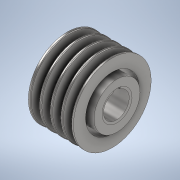
# Autodesk Inventor part: Polia Motora 3D
Saved by Autodesk Inventor 2021 (Build 250183000, 183)
## iProperties
Created: 2021-03-22
Part Number: Polia Motora 3D
Material: Steel, Carbon
Document SubType Name: Modeling
Designer: mathe
Mass: 3334.35 g
Surface Area: 1037.05 cm^2
Volume: 424.758 cm^3
Density: 7.85 g/cm^3
Appearance: Semi-Polished
Author: mathe
Autodesk Inventor part; units mm, degrees
ref_plane "YZ Plane" through (0, 0, 0) normal (1, 0, 0) x (0, 1, 0)
ref_plane "XZ Plane" through (0, 0, 0) normal (0, 1, 0) x (-1, 0, 0)
ref_plane "XY Plane" through (0, 0, 0) normal (0, 0, 1) x (1, 0, 0)
sketch "Sketch1" plane through (0, 0, 0) normal (0, 0, 1) x (1, 0, 0)
  arc A0 (466.2251, 430.0149) -> (467.1814, 430.7225) centre (466.2251, 431.0149) ccw
  arc A1 (466.2251, 430.0149) -> (467.1814, 430.7225) centre (466.2251, 431.0149) ccw
  arc A2 (478.0277, 430.7225) -> (478.984, 430.0149) centre (478.984, 431.0149) ccw
  arc A3 (478.0277, 430.7225) -> (478.984, 430.0149) centre (478.984, 431.0149) ccw
  line L0 (478.984, 430.0149) -> (482.1051, 430.0149)
  line L1 (478.984, 430.0149) -> (482.1051, 430.0149)
  line L2 (463.104, 430.0149) -> (466.2251, 430.0149)
  line L3 (463.104, 430.0149) -> (466.2251, 430.0149)
  arc A4 (482.1051, 430.0149) -> (483.0614, 430.7225) centre (482.1051, 431.0149) ccw
  arc A5 (482.1051, 430.0149) -> (483.0614, 430.7225) centre (482.1051, 431.0149) ccw
  arc A6 (462.1477, 430.7225) -> (463.104, 430.0149) centre (463.104, 431.0149) ccw
  arc A7 (462.1477, 430.7225) -> (463.104, 430.0149) centre (463.104, 431.0149) ccw
  line L4 (490.0745, 430.0149) -> (490.0745, 425.0149)
  line L5 (490.0745, 425.0149) -> (461.1309, 425.0149)
  line L6 (490.0745, 443.0149) -> (490.0745, 430.0149)
  line L7 (487.5595, 443.0149) -> (490.0745, 443.0149)
  line L8 (487.5595, 443.0149) -> (490.0745, 443.0149)
  line L9 (486.6032, 442.3073) -> (483.0614, 430.7225)
  line L10 (486.6032, 442.3073) -> (483.0614, 430.7225)
  line L11 (474.4859, 442.3073) -> (478.0277, 430.7225)
  line L12 (474.4859, 442.3073) -> (478.0277, 430.7225)
  line L13 (470.7232, 442.3073) -> (467.1814, 430.7225)
  line L14 (470.7232, 442.3073) -> (467.1814, 430.7225)
  arc A8 (471.6795, 443.0149) -> (470.7232, 442.3073) centre (471.6795, 442.0149) ccw
  arc A9 (471.6795, 443.0149) -> (470.7232, 442.3073) centre (471.6795, 442.0149) ccw
  line L15 (471.6795, 443.0149) -> (473.5296, 443.0149)
  line L16 (471.6795, 443.0149) -> (473.5296, 443.0149)
  arc A10 (474.4859, 442.3073) -> (473.5296, 443.0149) centre (473.5296, 442.0149) ccw
  arc A11 (474.4859, 442.3073) -> (473.5296, 443.0149) centre (473.5296, 442.0149) ccw
  arc A12 (453.1309, 419.5149) -> (454.1309, 420.5149) centre (453.1309, 420.5149) ccw
  arc A13 (460.1309, 420.5149) -> (461.1309, 419.5149) centre (461.1309, 420.5149) ccw
  line L17 (454.1309, 424.0149) -> (454.1309, 420.5149)
  arc A14 (461.1309, 425.0149) -> (460.1309, 424.0149) centre (461.1309, 424.0149) ccw
  arc A15 (454.1309, 424.0149) -> (453.1309, 425.0149) centre (453.1309, 424.0149) ccw
  line L18 (418.1309, 404.5149) -> (417.1309, 407.7149)
  line L19 (417.1309, 419.5149) -> (453.1309, 419.5149)
  line L20 (453.1309, 425.0149) -> (423.3745, 425.0149)
  arc A16 (434.4651, 430.0149) -> (435.4214, 430.7225) centre (434.4651, 431.0149) ccw
  arc A17 (434.4651, 430.0149) -> (435.4214, 430.7225) centre (434.4651, 431.0149) ccw
  arc A18 (430.3877, 430.7225) -> (431.344, 430.0149) centre (431.344, 431.0149) ccw
  arc A19 (430.3877, 430.7225) -> (431.344, 430.0149) centre (431.344, 431.0149) ccw
  line L21 (460.1309, 420.5149) -> (460.1309, 424.0149)
  line L22 (490.0745, 341.0149) -> (490.0745, 346.0149)
  line L23 (490.0745, 328.0149) -> (490.0745, 341.0149)
  arc A20 (483.0614, 340.3073) -> (482.1051, 341.0149) centre (482.1051, 340.0149) ccw
  arc A21 (483.0614, 340.3073) -> (482.1051, 341.0149) centre (482.1051, 340.0149) ccw
  line L24 (487.5595, 328.0149) -> (490.0745, 328.0149)
  line L25 (487.5595, 328.0149) -> (490.0745, 328.0149)
  arc A22 (486.6032, 328.7225) -> (487.5595, 328.0149) centre (487.5595, 329.0149) ccw
  arc A23 (486.6032, 328.7225) -> (487.5595, 328.0149) centre (487.5595, 329.0149) ccw
  line L26 (478.984, 341.0149) -> (482.1051, 341.0149)
  line L27 (478.984, 341.0149) -> (482.1051, 341.0149)
  arc A24 (478.984, 341.0149) -> (478.0277, 340.3073) centre (478.984, 340.0149) ccw
  arc A25 (478.984, 341.0149) -> (478.0277, 340.3073) centre (478.984, 340.0149) ccw
  line L28 (486.6032, 328.7225) -> (483.0614, 340.3073)
  line L29 (486.6032, 328.7225) -> (483.0614, 340.3073)
  line L30 (474.4859, 328.7225) -> (478.0277, 340.3073)
  line L31 (474.4859, 328.7225) -> (478.0277, 340.3073)
  arc A26 (473.5296, 328.0149) -> (474.4859, 328.7225) centre (473.5296, 329.0149) ccw
  arc A27 (473.5296, 328.0149) -> (474.4859, 328.7225) centre (473.5296, 329.0149) ccw
  line L32 (471.6795, 328.0149) -> (473.5296, 328.0149)
  line L33 (471.6795, 328.0149) -> (473.5296, 328.0149)
  arc A28 (470.7232, 328.7225) -> (471.6795, 328.0149) centre (471.6795, 329.0149) ccw
  arc A29 (470.7232, 328.7225) -> (471.6795, 328.0149) centre (471.6795, 329.0149) ccw
  line L34 (490.0745, 346.0149) -> (461.1309, 346.0149)
  line L35 (460.1309, 350.5149) -> (460.1309, 347.0149)
  arc A30 (460.1309, 347.0149) -> (461.1309, 346.0149) centre (461.1309, 347.0149) ccw
  line L36 (461.1309, 351.5149) -> (497.1309, 351.5149)
  arc A31 (453.1309, 346.0149) -> (454.1309, 347.0149) centre (453.1309, 347.0149) ccw
  arc A32 (438.9632, 328.7225) -> (439.9195, 328.0149) centre (439.9195, 329.0149) ccw
  arc A33 (438.9632, 328.7225) -> (439.9195, 328.0149) centre (439.9195, 329.0149) ccw
  line L37 (439.9195, 328.0149) -> (441.7696, 328.0149)
  line L38 (439.9195, 328.0149) -> (441.7696, 328.0149)
  arc A34 (441.7696, 328.0149) -> (442.7259, 328.7225) centre (441.7696, 329.0149) ccw
  arc A35 (441.7696, 328.0149) -> (442.7259, 328.7225) centre (441.7696, 329.0149) ccw
  line L39 (442.7259, 328.7225) -> (446.2677, 340.3073)
  arc A36 (447.224, 341.0149) -> (446.2677, 340.3073) centre (447.224, 340.0149) ccw
  arc A37 (447.224, 341.0149) -> (446.2677, 340.3073) centre (447.224, 340.0149) ccw
  line L40 (447.224, 341.0149) -> (450.3451, 341.0149)
  line L41 (447.224, 341.0149) -> (450.3451, 341.0149)
  arc A38 (451.3014, 340.3073) -> (450.3451, 341.0149) centre (450.3451, 340.0149) ccw
  arc A39 (451.3014, 340.3073) -> (450.3451, 341.0149) centre (450.3451, 340.0149) ccw
  line L42 (454.1309, 347.0149) -> (454.1309, 350.5149)
  line L43 (454.8432, 328.7225) -> (451.3014, 340.3073)
  line L44 (454.8432, 328.7225) -> (451.3014, 340.3073)
  line L45 (442.7259, 328.7225) -> (446.2677, 340.3073)
  line L46 (453.1309, 346.0149) -> (423.3745, 346.0149)
  line L47 (438.9632, 328.7225) -> (435.4214, 340.3073)
  line L48 (438.9632, 328.7225) -> (435.4214, 340.3073)
  arc A40 (435.4214, 340.3073) -> (434.4651, 341.0149) centre (434.4651, 340.0149) ccw
  line L49 (431.344, 341.0149) -> (434.4651, 341.0149)
  line L50 (431.344, 341.0149) -> (434.4651, 341.0149)
  arc A41 (431.344, 341.0149) -> (430.3877, 340.3073) centre (431.344, 340.0149) ccw
  arc A42 (431.344, 341.0149) -> (430.3877, 340.3073) centre (431.344, 340.0149) ccw
  line L51 (426.8459, 328.7225) -> (430.3877, 340.3073)
  line L52 (426.8459, 328.7225) -> (430.3877, 340.3073)
  arc A43 (425.8896, 328.0149) -> (426.8459, 328.7225) centre (425.8896, 329.0149) ccw
  arc A44 (425.8896, 328.0149) -> (426.8459, 328.7225) centre (425.8896, 329.0149) ccw
  line L53 (423.3745, 328.0149) -> (425.8896, 328.0149)
  line L54 (423.3745, 328.0149) -> (425.8896, 328.0149)
  line L55 (423.3745, 328.0149) -> (423.3745, 346.0149)
  arc A45 (435.4214, 340.3073) -> (434.4651, 341.0149) centre (434.4651, 340.0149) ccw
  line L56 (418.1309, 404.5149) -> (418.1309, 366.5149)
  line L57 (418.1309, 366.5149) -> (417.1309, 365.5149)
  line L58 (496.1309, 404.5149) -> (418.1309, 404.5149)
  line L59 (497.1309, 407.7149) -> (417.1309, 407.7149)
  line L60 (417.1309, 419.5149) -> (417.1309, 351.5149)
  line L61 (417.1309, 351.5149) -> (453.1309, 351.5149)
  line L62 (418.1309, 366.5149) -> (496.1309, 366.5149)
  line L63 (461.1309, 419.5149) -> (497.1309, 419.5149)
  line L64 (496.1309, 404.5149) -> (497.1309, 407.7149)
  arc A46 (454.1309, 350.5149) -> (453.1309, 351.5149) centre (453.1309, 350.5149) ccw
  line L65 (496.1309, 366.5149) -> (496.1309, 404.5149)
  line L66 (497.1309, 366.5149) -> (497.1309, 404.5149)
  line L67 (497.1309, 351.5149) -> (497.1309, 419.5149)
  line L68 (496.1309, 366.5149) -> (497.1309, 365.5149)
  arc A47 (461.1309, 351.5149) -> (460.1309, 350.5149) centre (461.1309, 350.5149) ccw
  arc A48 (454.8432, 328.7225) -> (455.7995, 328.0149) centre (455.7995, 329.0149) ccw
  arc A49 (454.8432, 328.7225) -> (455.7995, 328.0149) centre (455.7995, 329.0149) ccw
  line L69 (455.7995, 328.0149) -> (457.6496, 328.0149)
  line L70 (455.7995, 328.0149) -> (457.6496, 328.0149)
  arc A50 (457.6496, 328.0149) -> (458.6059, 328.7225) centre (457.6496, 329.0149) ccw
  arc A51 (457.6496, 328.0149) -> (458.6059, 328.7225) centre (457.6496, 329.0149) ccw
  arc A52 (487.5595, 443.0149) -> (486.6032, 442.3073) centre (487.5595, 442.0149) ccw
  arc A53 (487.5595, 443.0149) -> (486.6032, 442.3073) centre (487.5595, 442.0149) ccw
  line L71 (442.7259, 442.3073) -> (446.2677, 430.7225)
  line L72 (454.8432, 442.3073) -> (451.3014, 430.7225)
  line L73 (458.6059, 442.3073) -> (462.1477, 430.7225)
  arc A54 (458.6059, 442.3073) -> (457.6496, 443.0149) centre (457.6496, 442.0149) ccw
  arc A55 (455.7995, 443.0149) -> (454.8432, 442.3073) centre (455.7995, 442.0149) ccw
  line L74 (455.7995, 443.0149) -> (457.6496, 443.0149)
  arc A56 (442.7259, 442.3073) -> (441.7696, 443.0149) centre (441.7696, 442.0149) ccw
  line L75 (439.9195, 443.0149) -> (441.7696, 443.0149)
  line L76 (458.6059, 442.3073) -> (462.1477, 430.7225)
  arc A57 (458.6059, 442.3073) -> (457.6496, 443.0149) centre (457.6496, 442.0149) ccw
  arc A58 (455.7995, 443.0149) -> (454.8432, 442.3073) centre (455.7995, 442.0149) ccw
  line L77 (454.8432, 442.3073) -> (451.3014, 430.7225)
  arc A59 (450.3451, 430.0149) -> (451.3014, 430.7225) centre (450.3451, 431.0149) ccw
  arc A60 (450.3451, 430.0149) -> (451.3014, 430.7225) centre (450.3451, 431.0149) ccw
  line L78 (447.224, 430.0149) -> (450.3451, 430.0149)
  line L79 (447.224, 430.0149) -> (450.3451, 430.0149)
  arc A61 (446.2677, 430.7225) -> (447.224, 430.0149) centre (447.224, 431.0149) ccw
  arc A62 (446.2677, 430.7225) -> (447.224, 430.0149) centre (447.224, 431.0149) ccw
  line L80 (442.7259, 442.3073) -> (446.2677, 430.7225)
  arc A63 (442.7259, 442.3073) -> (441.7696, 443.0149) centre (441.7696, 442.0149) ccw
  line L81 (439.9195, 443.0149) -> (441.7696, 443.0149)
  line L82 (455.7995, 443.0149) -> (457.6496, 443.0149)
  line L83 (423.3745, 443.0149) -> (423.3745, 425.0149)
  line L84 (426.8459, 442.3073) -> (430.3877, 430.7225)
  arc A64 (439.9195, 443.0149) -> (438.9632, 442.3073) centre (439.9195, 442.0149) ccw
  line L85 (438.9632, 442.3073) -> (435.4214, 430.7225)
  arc A65 (426.8459, 442.3073) -> (425.8896, 443.0149) centre (425.8896, 442.0149) ccw
  line L86 (423.3745, 443.0149) -> (425.8896, 443.0149)
  line L87 (431.344, 430.0149) -> (434.4651, 430.0149)
  line L88 (426.8459, 442.3073) -> (430.3877, 430.7225)
  arc A66 (439.9195, 443.0149) -> (438.9632, 442.3073) centre (439.9195, 442.0149) ccw
  line L89 (438.9632, 442.3073) -> (435.4214, 430.7225)
  line L90 (423.3745, 443.0149) -> (425.8896, 443.0149)
  arc A67 (426.8459, 442.3073) -> (425.8896, 443.0149) centre (425.8896, 442.0149) ccw
  line L91 (431.344, 430.0149) -> (434.4651, 430.0149)
  line L92 (458.6059, 328.7225) -> (462.1477, 340.3073)
  line L93 (470.7232, 328.7225) -> (467.1814, 340.3073)
  arc A68 (467.1814, 340.3073) -> (466.2251, 341.0149) centre (466.2251, 340.0149) ccw
  arc A69 (467.1814, 340.3073) -> (466.2251, 341.0149) centre (466.2251, 340.0149) ccw
  line L94 (463.104, 341.0149) -> (466.2251, 341.0149)
  line L95 (463.104, 341.0149) -> (466.2251, 341.0149)
  arc A70 (463.104, 341.0149) -> (462.1477, 340.3073) centre (463.104, 340.0149) ccw
  arc A71 (463.104, 341.0149) -> (462.1477, 340.3073) centre (463.104, 340.0149) ccw
  line L96 (458.6059, 328.7225) -> (462.1477, 340.3073)
  line L97 (470.7232, 328.7225) -> (467.1814, 340.3073)
  line L98 (416.3181, 385.5149) -> (497.1309, 385.5149)
  point P0 (0, 0)
  dimension "d1" = 1
  dimension "d3" = 38
  dimension "d5" = 68
  dimension "d7" = 1
  dimension "d9" = 34
  dimension "d11" = 13
  constraints: 198 end point, 144 point on circle, 72 centre point, 6 point on line
  measures "d1" radius of A14
  measures "d3" distance of L56.end L18.start
  measures "d5" distance of L19.start L60.end
  measures "d7" radius of A15
  measures "d9" angle of L89 L88
  measures "d11" distance from line of L83.start L87
revolve "Revolution1" add sketch "Sketch1" angle 360 about axis through (416.3181, 385.5149, 0) along (1, 0, 0) contours A0 L13 A8 L15 A10 L11 A2 L0 A4 L9 A52 L7 L6 L4 L5 A14 L21 A13 L63 L67 L59 L60 L19 A12 L17 A15 L20 L83 L86 A65 L84 A18 L87 A16 L85 A64 L75 A56 L71 A61 L78 A59 L72 A55 L74 A54 L73 A6 L2 | L64 L58 L18 L59
sketch "Sketch2" plane through (417.1309, 385.5149, 0) normal (-1, 0, 0) x (0, 0, 1)
  circle A0 centre (0, 0) radius 19 projected
  line L0 (0, 19) -> (0, 22.2)
  line L1 (0, 22.2) -> (5, 22.2)
  circle A1 centre (0, 0) radius 22.2 projected
  line L2 (5, 22.2) -> (5, 18.3303)
  line L3 (0, 22.2) -> (-5, 22.2)
  line L4 (-5, 22.2) -> (-5, 18.3303)
  point P0 (0, -385.5149)
  point P1 (5, 21.6296)
  point P2 (-5, 21.6296)
  dimension "d13" = 3.2
  dimension "d14" = 5
  constraints: 10 end point, 3 horizontal, 3 point on circle, 2 perpendicular, 1 vertical, 1 other
  measures "d13" distance of L0.start L0.end
  measures "d14" distance of L0.end L3.end
extrude "Extrusion1" cut sketch "Sketch2" against normal through all contours A0 L0 A1 L2 | L4 A1 L0 A0
body "Solid1"
